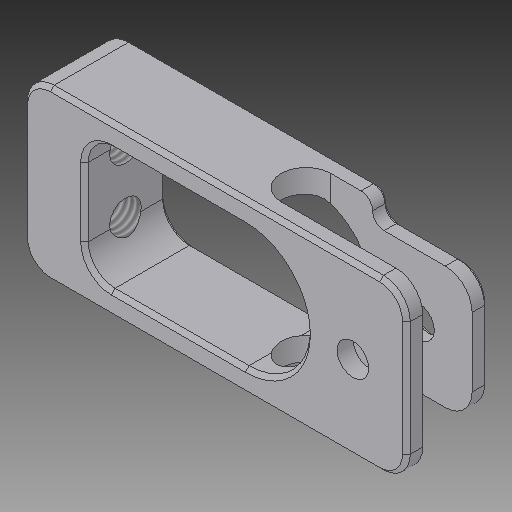
# Autodesk Inventor part: Coulisse
Saved by Autodesk Inventor 2017 (Build 210142000, 142)
## iProperties
Company: FABLAB Fenchmakers
Part Number: Coulisse
Material: ----------
Document SubType Name: Modeling
Designer: FABLAB Frenchmakers
Density: 7.86 g/cm^3
Appearance: Métal - Acier
Mass: 33.3632 g
Surface Area: 37.0241 cm^2
Volume: 4.24468 cm^3
Project: 1420 Vauban 3D XL
Catalog Web Link: http://frenchmakers.com/
Stock Number: 1420-05-15
Autodesk Inventor part; units mm, degrees
ref_plane "YZ Plane" through (0, 0, 0) normal (1, 0, 0) x (0, 1, 0)
ref_plane "XZ Plane" through (0, 0, 0) normal (0, 1, 0) x (-1, 0, 0)
ref_plane "XY Plane" through (0, 0, 0) normal (0, 0, 1) x (1, 0, 0)
sketch "Esquisse1" plane through (0, 0, 0) normal (0, 0, 1) x (1, 0, 0)
  line L0 (-25, -11) -> (25, -11)
  line L1 (25, -11) -> (25, 11)
  line L2 (25, 11) -> (-25, 11)
  line L3 (-25, 11) -> (-25, -11)
  line L4 (-25, -11) -> (25, 11) construction
  line L5 (25, -11) -> (-25, 11) construction
  point P0 (0, 0)
  dimension "d0" = 50
  dimension "d1" = 22
  constraints: 12 end point, 2 midpoint, 2 parallel, 1 horizontal, 1 perpendicular
  measures "d0" distance between parallel lines of L1 L3
  measures "d1" distance between parallel lines of L0 L2
extrude "Extrusion1" add sketch "Esquisse1" along normal mid plane 10.7
fillet "Congé1" radius 3.5 4 edges at (-25, 11, 0) (-25, -11, 0) (25, 11, 0) (25, -11, 0)
sketch "Esquisse2" plane through (0, 0, 5.35) normal (0, 0, 1) x (1, 0, 0)
  line L0 (-13.55, -8) -> (3.95, -8)
  line L1 (3.95, 8) -> (-13.55, 8)
  line L2 (-17.05, 4.5) -> (-17.05, -4.5)
  arc A0 (3.95, -8) -> (3.95, 8) centre (3.95, 0) ccw
  line L3 (-25, 7.5) -> (-25, -7.5) projected
  arc A1 (-13.55, 8) -> (-17.05, 4.5) centre (-13.55, 4.5) ccw
  arc A2 (-17.05, -4.5) -> (-13.55, -8) centre (-13.55, -4.5) ccw
  point P0 (0, 0)
  point P1 (-17.05, 0)
  dimension "d5" = 16
  dimension "d6" = 21
  dimension "d7" = 7.95
  dimension "d8" = 3.5
  constraints: 6 end point, 6 point on circle, 6 tangent, 3 centre point, 1 equal radius, 1 horizontal, 1 horizontal alignment, 1 midpoint, 1 parallel
  measures "d5" distance between parallel lines of L0 L1
  measures "d6" distance from line of A0.centre L2
  measures "d7" distance between parallel lines of L3 L2
  measures "d8" radius of A1
extrude "Extrusion2" cut sketch "Esquisse2" against normal through all
sketch "Esquisse3" plane through (-21.5, 11, -5.35) normal (0, 1, 0) x (1, 0, 0)
  line L0 (28.025, -8.575) -> (46.5, -8.575)
  line L1 (46.5, -8.575) -> (46.5, -2.125)
  line L2 (46.5, -2.125) -> (28.025, -2.125)
  arc A0 (28.025, -2.125) -> (28.025, -8.575) centre (28.025, -5.35) ccw
  line L3 (-3.5, 0) -> (-3.5, -10.7) projected
  line L4 (46.5, -10.7) -> (46.5, 0) projected
  point P0 (21.5, -5.35)
  dimension "d11" = 6.45
  dimension "d13" = 28.3
  constraints: 6 end point, 2 point on circle, 2 tangent, 1 centre point, 1 collinear, 1 horizontal, 1 horizontal alignment, 1 parallel, 1 perpendicular
  measures "d11" distance between parallel lines of L2 L0
  measures "d13" distance edge to line of A0 L3
extrude "Extrusion3" cut sketch "Esquisse3" against normal through all
sketch "Esquisse4" plane through (-25, -7.5, 5.35) normal (-1, 0, 0) x (0, 0, 1)
  point P0 (-5.35, 7.5)
  point P1 (-5.35, 3.475)
  point P2 (-5.35, 11.525)
  dimension "d16" = 8.05
  dimension "d17" = 4.025
  constraints: 2 vertical alignment
  measures "d16" distance of point (-5.35, 11.525) point (-5.35, 3.475)
  measures "d17" distance of point (-5.35, 7.5) point (-5.35, 11.525)
hole "Perçage1" at (-25, -4.025, 0) at (-25, 4.025, 0) direction (1, 0, 0) diameter 4.134 depth 14.2 tip angle 118 thread size "M5x0.8" class "6H" standard "ISO Metric profile"
sketch "Esquisse5" plane through (0, 0, -5.35) normal (0, 0, -1) x (-1, 0, 0)
  line L0 (-25, 7.5) -> (-25, -7.5) projected
  point P0 (0, 0)
  point P1 (-18, 0)
  dimension "d25" = 7
  constraints: 1 horizontal alignment
  measures "d25" distance from line of L0 point (-18, 0)
hole "Perçage2" at (18, 0, -5.35) direction (0, 0, 1) diameter 4.134 end through all
sketch "Esquisse6" plane through (0, 0, -5.35) normal (0, 0, -1) x (-1, 0, 0)
  line L0 (-12, -8) -> (-25, -8)
  line L1 (-25, -8) -> (-25, -11)
  line L2 (-25, -11) -> (-12, -11)
  line L3 (-12, -11) -> (-12, -8)
  line L4 (-12, 11) -> (-25, 11)
  line L5 (-25, 11) -> (-25, 8)
  line L6 (-25, 8) -> (-12, 8)
  line L7 (-12, 8) -> (-12, 11)
  line L8 (-21.5, -11) -> (21.5, -11) projected
  line L9 (21.5, 11) -> (-21.5, 11) projected
  line L10 (-25, 7.5) -> (-25, -7.5) projected
  line L11 (25, -7.5) -> (25, 7.5) projected
  point P0 (0, 0)
  dimension "d33" = 16
  dimension "d34" = 8
  dimension "d36" = 13
  constraints: 16 end point, 5 collinear, 4 parallel, 2 horizontal, 2 perpendicular
  measures "d33" distance between parallel lines of L6 L0
  measures "d34" distance from line of point (0, 0) L0
  measures "d36" distance between parallel lines of L1 L3
extrude "Extrusion4" cut sketch "Esquisse6" against normal up to surface (2.125 mm away)
fillet "Congé2" radius 3.5 2 edges at (24.9641, -8, -4.2875) (24.9641, 8, -4.2875)
fillet "Congé3" radius 1.5 4 edges at (12, -8, -4.2875) (12, -11, -4.2875) (12, 11, -4.2875) (12, 8, -4.2875)
chamfer "Chanfrein1" distance 0.75 angle 45 1 edges at (18, -2.067, -5.35)
chamfer "Chanfrein2" distance 0.5 angle 45 34 edges at (-4.8, -8, -5.35) (11.95, 0, -5.35) (-4.8, 8, -5.35) (-16.0249, 6.9749, -5.35) (-17.05, 0, -5.35) (-16.0249, -6.9749, -5.35) (11.95, 0, 5.35) (-4.8, -8, 5.35) (-16.0249, -6.9749, 5.35) (-17.05, 0, 5.35) (-16.0249, 6.9749, 5.35) (-4.8, 8, 5.35) (-23.9749, -9.9749, -5.35) (-5.4999, -11, -5.35) (11.5607, -10.5607, -5.35) (12.4393, -8.4393, -5.35) (17.5, -8, -5.35) (23.9749, -6.9749, -5.35) (25, 0, -5.35) (23.9749, 6.9749, -5.35) (17.5, 8, -5.35) (12.4393, 8.4393, -5.35) (11.5607, 10.5607, -5.35) (-5.4999, 11, -5.35) (-23.9749, 9.9749, -5.35) (-25, 0, -5.35) (-23.9749, -9.9749, 5.35) (-25, 0, 5.35) (-23.9749, 9.9749, 5.35) (0, 11, 5.35) (23.9749, 9.9749, 5.35) (25, 0, 5.35) (23.9749, -9.9749, 5.35) (0, -11, 5.35)
equation "\"d17\" = 0.5 * d16"
equation "\"d34\" = 0.5 * d33"
